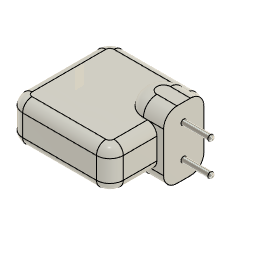
charger v1 (Autodesk Fusion 360 design; units mm, degrees)
Autodesk Fusion 360 part; units mm, degrees
sketch "Sketch1" plane through (0, 0, 0) normal (0, 0, 1) x (1, 0, 0)
  line L0 (-10, 0) -> (-65, 0)
  line L1 (-75, 10) -> (-75, 65)
  line L2 (-65, 75) -> (-10, 75)
  line L3 (0, 65) -> (0, 10)
  arc A0 (-10, 0) -> (0, 10) centre (-10, 10) ccw
  arc A1 (-75, 10) -> (-65, 0) centre (-65, 10) ccw
  arc A2 (-65, 75) -> (-75, 65) centre (-65, 65) ccw
  arc A3 (0, 65) -> (-10, 75) centre (-10, 65) ccw
  dimension "d1" = 10
  constraint horizontal L0
  constraint vertical L1
  constraint horizontal L2
  constraint vertical L3
  constraint tangent L0 A0
  constraint tangent L3 A0
  constraint tangent L0 A1
  constraint tangent L1 A1
  constraint equal A0 A1
  constraint tangent L1 A2
  constraint tangent L2 A2
  constraint equal A0 A2
  constraint tangent L2 A3
  constraint tangent L3 A3
  constraint equal A0 A3
  measures "d1" radius of A0
extrude "Extrude1" add sketch "Sketch1" along normal mid plane 30 makes body 1
sketch "Sketch3" plane through (0, 0, 15) normal (0, 0, 1) x (-1, 0, 0)
  arc A0 (10, 0) -> (0, -10) centre (10, -10) ccw
  line L0 (0, -10) -> (0, -65)
  arc A1 (0, -65) -> (10, -75) centre (10, -65) ccw
  line L1 (10, -75) -> (65, -75)
  arc A2 (65, -75) -> (75, -65) centre (65, -65) ccw
  line L2 (75, -65) -> (75, -10)
  arc A3 (75, -10) -> (65, 0) centre (65, -10) ccw
  line L3 (65, 0) -> (10, 0)
  line L4 (10, -65) -> (0, -65)
  line L5 (10, -35) -> (0, -35)
  line L6 (0, -35) -> (0, -65)
  arc A4 (10, -65) -> (10, -35) centre (10, -50) ccw
  constraint coincident L0 A1.start
  constraint tangent L4 A4
  constraint perpendicular L0 L4
  constraint tangent L5 A4
  constraint perpendicular L0 L5
  constraint perpendicular L4 L6
extrude "Extrude4" cut sketch "Sketch3" against normal blind 45 contours L0 L4 L5 L6 A4 bodies 1
extrude "Extrude5" add sketch "Sketch3" along normal blind 10 and the other way blind 40 separate body contours L0 L4 L5 L6 A4 makes body 2
fillet "Fillet2" radius 10 3 edges at (-5, 65, 25) (-25, 50, 25) (-5, 35, 25) on bodies 2
fillet "Fillet3" radius 10 3 edges at (-5, 35, -25) (-25, 50, -25) (-5, 65, -25) on bodies 2
extrude "Extrude6" add 1 faces at (0, 45, -5) along direction (1, 0, 0) blind 5 on bodies 2 bodies 2
sketch "Sketch4" plane through (5, 0, 0) normal (1, 0, 0) x (0, 1, 0)
  arc A0 (55, -25) -> (65, -15) centre (55, -15) ccw
  line L0 (65, -15) -> (65, 15)
  arc A1 (65, 15) -> (55, 25) centre (55, 15) ccw
  line L1 (55, 25) -> (45, 25)
  arc A2 (45, 25) -> (35, 15) centre (45, 15) ccw
  line L2 (35, 15) -> (35, -15)
  arc A3 (35, -15) -> (45, -25) centre (45, -15) ccw
  line L3 (45, -25) -> (55, -25)
  circle A4 centre (50, 12) radius 2
  circle A5 centre (50, -12) radius 2
extrude "Extrude7" add sketch "Sketch4" along normal blind 22 separate body contours A4 | A5 makes body 3 at (19.6667, 50.637, 13.8959) makes body 4 at (19.6667, 50.637, -10.1041)
fillet "Fillet4" radius 2 2 edges at (27, 48.1353, 11.2768) (27, 48.1353, -12.7232) on bodies 3 4
fillet "Fillet5" radius 7 16 edges at (-2.9289, 72.0711, 15) (-37.5, 75, 15) (-72.0711, 72.0711, 15) (-75, 37.5, 15) (-72.0711, 2.9289, 15) (-37.5, 0, 15) (-2.9289, 2.9289, 15) (0, 22.5, 15) (0, 22.5, -15) (-2.9289, 2.9289, -15) (-37.5, 0, -15) (-72.0711, 2.9289, -15) (-75, 37.5, -15) (-72.0711, 72.0711, -15) (-37.5, 75, -15) (-2.9289, 72.0711, -15) on bodies 1
sketch "Sketch5" plane through (-75, 0, 0) normal (-1, 0, 0) x (0, -1, 0)
  line L0 (-65, -8) -> (-10, -8)
  line L1 (-10, -8) -> (-10, 8)
  line L2 (-10, 8) -> (-65, 8)
  line L3 (-65, 8) -> (-65, -8)
  line L4 (-56, 7) -> (-49, 7)
  line L5 (-49, 7) -> (-49, -7)
  line L6 (-49, -7) -> (-56, -7)
  line L7 (-56, -7) -> (-56, 7)
  constraint horizontal L4
  constraint vertical L5
  constraint horizontal L6
  constraint vertical L7
extrude "Extrude8" cut sketch "Sketch5" against normal blind 10 contours L4 L5 L6 L7 bodies 1
sketch "Sketch6" plane through (-65, 0, 0) normal (-1, 0, 0) x (0, -1, 0)
  line L0 (-56, -7) -> (-49, -7)
  line L1 (-49, -7) -> (-49, 7)
  line L2 (-49, 7) -> (-56, 7)
  line L3 (-56, 7) -> (-56, -7)
  line L4 (-50.5, 6.5) -> (-51.5, 6.5)
  line L5 (-51.5, 6.5) -> (-51.5, -6.5)
  line L6 (-51.5, -6.5) -> (-50.5, -6.5)
  line L7 (-50.5, -6.5) -> (-50.5, 6.5)
  constraint horizontal L4
  constraint vertical L5
  constraint horizontal L6
  constraint vertical L7
extrude "Extrude9" add sketch "Sketch6" along normal blind 10 contours L4 L5 L6 L7 bodies 1
extrude "Extrude10" cut 1 faces at (-75, 51.1667, 2.1667) along direction (1, 0, 0) blind 2 on bodies 1 bodies 1
